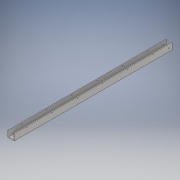
# Autodesk Inventor part: 1x1 U-Channel
Saved by Autodesk Inventor 2018 (Build 220112000, 112)
## iProperties
Created: 2019-01-19
Part Number: 1x1 U-Channel
Material: Generic
Document SubType Name: Modeling
Designer: maste
Density: 1 g/cm^3
Appearance: Default
Author: maste
Autodesk Inventor part; units mm, degrees
ref_plane "YZ Plane" through (0, 0, 0) normal (1, 0, 0) x (0, 1, 0)
ref_plane "XZ Plane" through (0, 0, 0) normal (0, 1, 0) x (-1, 0, 0)
ref_plane "XY Plane" through (0, 0, 0) normal (0, 0, 1) x (1, 0, 0)
sketch "Sketch1" plane through (0, 0, 0) normal (0, 0, 1) x (1, 0, 0)
  line L0 (0, 0) -> (25.4, 0)
  line L1 (25.4, 0) -> (25.4, 25.4)
  line L2 (25.4, 25.4) -> (0, 25.4)
  line L3 (0, 25.4) -> (0, 0)
  line L4 (3.175, 22.225) -> (22.225, 22.225)
  line L5 (22.225, 22.225) -> (22.225, 3.175)
  line L6 (22.225, 3.175) -> (3.175, 3.175)
  line L7 (3.175, 3.175) -> (3.175, 22.225)
  dimension "d0" = 25.4
  dimension "d1" = 25.4
  dimension "d2" = 3.175
  constraints: 16 end point, 4 parallel, 2 perpendicular, 1 horizontal, 3 other
  measures "d0" distance of L2.end L1.end
  measures "d1" distance of L1.end L0.end
  measures "d2" distance between parallel lines of L2 L4
extrude "Extrusion1" add sketch "Sketch1" along normal blind 635
sketch "Sketch2" plane through (25.4, 0, 0) normal (1, 0, 0) x (0, 0, -1)
  line L0 (0, 0) -> (0, 25.4) construction
  line L1 (0, 25.4) -> (0, 18.7198) construction
  line L2 (0, 25.4) -> (0, 21.7678) construction
  line L3 (0, 22.225) -> (-635, 22.225) construction
  line L4 (0, 21.7678) -> (-76.2, 21.7678) construction
  line L5 (-76.2, 21.7678) -> (-177.8, 21.7678) construction
  line L6 (-177.8, 21.7678) -> (-279.4, 21.7678) construction
  line L7 (-279.4, 21.7678) -> (-381, 21.7678) construction
  line L8 (-381, 21.7678) -> (-482.6, 21.7678) construction
  line L9 (-482.6, 21.7678) -> (-584.2, 21.7678) construction
  circle A0 centre (-76.2, 21.7678) radius 1.3208
  circle A1 centre (-177.8, 21.7678) radius 1.3208
  circle A2 centre (-279.4, 21.7678) radius 1.3208
  circle A3 centre (-381, 21.7678) radius 1.3208
  circle A4 centre (-482.6, 21.7678) radius 1.3208
  circle A5 centre (-584.2, 21.7678) radius 1.3208
  dimension "d5" = 6.6802
  dimension "d6" = 3.6322
  dimension "d8" = 76.2
  dimension "d9" = 101.6
  dimension "d11" = 101.6
  dimension "d12" = 101.6
  dimension "d13" = 101.6
  dimension "d14" = 101.6
  dimension "d15" = 2.6416
  constraints: 16 end point, 6 centre point, 6 coincident, 5 point on line, 3 horizontal
  measures "d5" distance of L0.end L1.end
  measures "d6" distance of L0.end L2.end
  measures "d8" distance of L2.end L4.end
  measures "d9" distance of L4.end L5.end
  measures "d11" distance of L5.end L6.end
  measures "d12" distance of L6.end L7.end
  measures "d13" distance of L7.end L8.end
  measures "d14" distance of L8.end L9.end
  measures "d15" diameter of A0
extrude "Extrusion2" cut sketch "Sketch2" against normal blind 635
sketch "Sketch3" plane through (0, 0, 635) normal (0, 0, 1) x (1, 0, 0)
  line L0 (3.175, 3.175) -> (3.175, 22.225) projected
  line L1 (3.175, 22.225) -> (22.225, 22.225)
  line L2 (22.225, 22.225) -> (22.225, 42.4073)
  line L3 (22.225, 42.4073) -> (3.175, 42.4073)
  line L4 (3.175, 42.4073) -> (3.175, 22.225)
  point P0 (0, 0)
  dimension "d18" = 19.05
  constraints: 8 end point, 2 parallel, 1 horizontal, 1 perpendicular
  measures "d18" distance of L3.end L2.end
extrude "Extrusion3" cut sketch "Sketch3" against normal blind 635
sketch "Sketch4" plane through (25.4, 0, 0) normal (1, 0, 0) x (0, 0, -1)
  line L0 (0, 25.4) -> (0, 0) projected
  line L1 (0, 12.7) -> (-12.7, 12.7) construction
  line L2 (0, 12.7) -> (12.7, 12.7) construction
  circle A0 centre (-12.7, 12.7) radius 2.5797
  dimension "d21" = 12.7
  dimension "d22" = 180
  dimension "d23" = 5.1594
  constraints: 4 end point, 2 horizontal, 1 centre point, 1 coincident, 1 collinear, 1 midpoint
  measures "d21" distance of L1.start L1.end
  measures "d22" angle of L1 L2
  measures "d23" diameter of A0
extrude "Extrusion4" cut sketch "Sketch4" against normal blind 635
sketch "Sketch5" plane through (0, 0, 0) normal (0, -1, 0) x (1, 0, 0)
  line L0 (0, 0) -> (25.4, 0) construction
  line L1 (12.7, 0) -> (12.7, 12.7) construction
  line L2 (12.7, 0) -> (25.4, 0) construction
  circle A0 centre (12.7, 12.7) radius 2.5797
  dimension "d26" = 12.7
  dimension "d27" = 90
  dimension "d28" = 5.1594
  constraints: 4 end point, 1 centre point, 1 coincident, 1 horizontal, 1 midpoint, 1 perpendicular, 1 vertical
  measures "d26" distance of L1.start L1.end
  measures "d27" angle of L2 L1
  measures "d28" diameter of A0
extrude "Extrusion6" cut sketch "Sketch5" against normal blind 635
body "Solid1"
